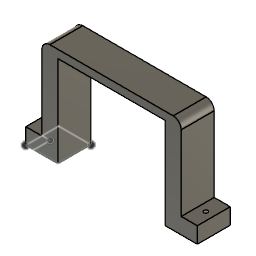
Bigger Clamp (Autodesk Fusion 360 design; units mm, degrees)
part number: 2026-02-06-17-12-58-600
Autodesk Fusion 360 part; units mm, degrees
sketch "Sketch1" plane through (0, 0, 0) normal (0, 1, 0) x (1, 0, 0)
  line L0 (0, 0) -> (66.6, 0)
  line L1 (66.6, 0) -> (66.6, -56.6)
  line L2 (66.6, -56.6) -> (0, -56.6)
  line L3 (0, -56.6) -> (0, 0)
  line L4 (0, 0) -> (-20, 0)
  line L5 (-20, 0) -> (-20, -10)
  line L6 (-20, -10) -> (-10, -10)
  line L7 (0, -10) -> (0, 0)
  line L8 (-10, -10) -> (-10, -66.6)
  line L9 (-10, -66.6) -> (0, -66.6)
  line L10 (0, -56.6) -> (0, -10)
  line L11 (0, -66.6) -> (66.6, -66.6)
  line L12 (66.6, -56.6) -> (0, -56.6)
  line L13 (66.6, -66.6) -> (76.6, -66.6)
  line L14 (76.6, -66.6) -> (76.6, -10)
  line L15 (76.6, 0) -> (66.6, 0)
  line L16 (66.6, 0) -> (66.6, -56.6)
  line L17 (66.6, 0) -> (86.6, 0)
  line L18 (86.6, 0) -> (86.6, -10)
  line L19 (86.6, -10) -> (76.6, -10)
  line L20 (66.6, -10) -> (66.6, 0)
  dimension "d19" = 66.6
  dimension "d20" = 56.6
  dimension "d21" = 20
  dimension "d22" = 10
  dimension "d23" = 10
  dimension "d24" = 56.6
  dimension "d25" = 10
  dimension "d26" = 20
  dimension "d27" = 10
  constraint horizontal L0
  constraint vertical L1
  constraint horizontal L2
  constraint vertical L3
  constraint coincident L0.start L3.end
  constraint horizontal L4
  constraint vertical L5
  constraint horizontal L6
  constraint vertical L7
  constraint vertical L8
  constraint horizontal L9
  constraint vertical L10
  constraint horizontal L11
  constraint horizontal L12
  constraint horizontal L13
  constraint vertical L14
  constraint horizontal L15
  constraint vertical L16
  constraint horizontal L17
  constraint vertical L18
  constraint horizontal L19
  constraint vertical L20
  measures "d19" distance of L0.start L0.end
  measures "d20" distance of L0.start L2.end
  measures "d21" distance of L0.start L4.end
  measures "d22" distance of L0.start L7.start
  measures "d23" distance of L7.start L6.end
  measures "d24" distance of L7.start L9.end
  measures "d25" distance of L11.end L13.end
  measures "d26" distance of L0.end L17.end
  measures "d27" distance of L0.end L20.start
extrude "Extrude2" add sketch "Sketch1" along normal blind 20.5 contours L1 L2 L3 L4 L5 L6 L7 L8 L9 L10 L11 L12 L13 L14 L15 L16 L17 L18 L19 L20
sketch "Sketch4" plane through (0, 0, 10) normal (0, 0, 1) x (-1, 0, 0)
  line L0 (20, 0) -> (10, 0)
  line L1 (10, 0) -> (10, -20.5)
  line L2 (10, -20.5) -> (20, -20.5)
  line L3 (20, -20.5) -> (20, 0)
  circle A0 centre (15, -10.25) radius 1.5
  dimension "d32" = 3
  measures "d32" diameter of A0
sketch "Sketch5" plane through (0, 0, 10) normal (0, 0, 1) x (-1, 0, 0)
  line L0 (-76.6, 0) -> (-86.6, 0)
  line L1 (-86.6, 0) -> (-86.6, -20.5)
  line L2 (-86.6, -20.5) -> (-76.6, -20.5)
  line L3 (-76.6, -20.5) -> (-76.6, 0)
  circle A0 centre (-81.6, -10.25) radius 1.5
  dimension "d33" = 3
  measures "d33" diameter of A0
hole "Hole2" at (-15, 10.25, 10) at (81.6, 10.25, 10) direction (0, 0, -1) diameter 2.529 depth 15 tip angle 118
thread "Thread2" "ISO Metric profile 3.0 M3x0.5 M3x0.5 6H" thread offset 0 thread depth 7.4
sketch "Sketch6" plane through (0, 0, 0) normal (0, 0, -1) x (1, 0, 0)
  circle A0 centre (-15, -10.25) radius 1.2645
  line L0 (0, 0) -> (-20, 0)
  line L1 (-20, 0) -> (-20, -20.5)
  line L2 (-20, -20.5) -> (0, -20.5)
  line L3 (0, -20.5) -> (0, 0)
  line L4 (-20, 0) -> (0, 0)
  line L5 (0, 0) -> (0, -20.5)
  line L6 (0, -20.5) -> (-20, -20.5)
  line L7 (-20, -20.5) -> (-20, 0)
  line L8 (-15, -10.25) -> (-20, -10.25)
  line L9 (-15, -10.25) -> (-15, 0)
  constraint horizontal L4
  constraint vertical L5
  constraint horizontal L6
  constraint vertical L7
  constraint coincident L2.end L3.start
  constraint coincident L0.end L1.start
  constraint coincident A0.centre L8.start
  constraint midpoint L1 L8.end
  constraint coincident L4 L9.end
  constraint perpendicular L4 L9
extrude "Extrude3" cut 1 faces at (18.8667, 6.8333, 66.6) along direction (0, 0, -1) blind 5
fillet "Fillet3" radius 5 2 edges at (-10, 10.25, 61.6) (76.6, 10.25, 61.6)
